Autodesk Fusion 360 part; units mm, degrees
(part 4 of 5)
  line L859 (16.6192, -17.6237) -> (17.4198, -17.6237)
  line L860 (17.4198, -17.6237) -> (17.4198, -20.7216)
  line L861 (17.4198, -20.7216) -> (16.6192, -20.7216)
  line L862 (16.6192, -20.7216) -> (16.6192, -21.722)
  line L863 (16.6192, -21.722) -> (2.6196, -21.722)
  line L864 (364.282, -27.7716) -> (365.083, -27.7716)
  line L865 (365.083, -27.7716) -> (365.083, -30.8722)
  line L866 (365.083, -30.8722) -> (364.282, -30.8722)
  line L867 (364.282, -30.8722) -> (364.282, -36.6737)
  line L868 (364.282, -36.6737) -> (365.083, -36.6737)
  line L869 (365.083, -36.6737) -> (365.083, -39.7715)
  line L870 (365.083, -39.7715) -> (364.282, -39.7715)
  line L871 (364.282, -39.7715) -> (364.282, -40.7719)
  line L872 (364.282, -40.7719) -> (350.282, -40.7719)
  line L873 (350.282, -40.7719) -> (350.282, -39.7715)
  line L874 (350.282, -39.7715) -> (349.481, -39.7715)
  line L875 (349.481, -39.7715) -> (349.481, -36.6737)
  line L876 (349.481, -36.6737) -> (350.282, -36.6737)
  line L877 (350.282, -36.6737) -> (350.282, -30.8722)
  line L878 (350.282, -30.8722) -> (349.481, -30.8722)
  line L879 (349.481, -30.8722) -> (349.481, -27.7716)
  line L880 (349.481, -27.7716) -> (350.282, -27.7716)
  line L881 (350.282, -27.7716) -> (350.282, -26.7725)
  line L882 (350.282, -26.7725) -> (364.282, -26.7725)
  line L883 (364.282, -26.7725) -> (364.282, -27.7716)
  line L884 (278.557, -39.7715) -> (278.557, -40.7719)
  line L885 (278.557, -40.7719) -> (264.557, -40.7719)
  line L886 (264.557, -40.7719) -> (264.557, -39.7715)
  line L887 (264.557, -39.7715) -> (263.756, -39.7715)
  line L888 (263.756, -39.7715) -> (263.756, -36.6737)
  line L889 (263.756, -36.6737) -> (264.557, -36.6737)
  line L890 (264.557, -36.6737) -> (264.557, -30.8722)
  line L891 (264.557, -30.8722) -> (263.756, -30.8722)
  line L892 (263.756, -30.8722) -> (263.756, -27.7716)
  line L893 (263.756, -27.7716) -> (264.557, -27.7716)
  line L894 (264.557, -27.7716) -> (264.557, -26.7725)
  line L895 (264.557, -26.7725) -> (278.557, -26.7725)
  line L896 (278.557, -26.7725) -> (278.557, -27.7716)
  line L897 (278.557, -27.7716) -> (279.356, -27.7716)
  line L898 (279.356, -27.7716) -> (279.356, -30.8722)
  line L899 (279.356, -30.8722) -> (278.557, -30.8722)
  line L900 (278.557, -30.8722) -> (278.557, -36.6737)
  line L901 (278.557, -36.6737) -> (279.356, -36.6737)
  line L902 (279.356, -36.6737) -> (279.356, -39.7715)
  line L903 (279.356, -39.7715) -> (278.557, -39.7715)
  line L904 (244.706, -36.6737) -> (245.507, -36.6737)
  line L905 (245.507, -36.6737) -> (245.507, -30.8722)
  line L906 (245.507, -30.8722) -> (244.706, -30.8722)
  line L907 (244.706, -30.8722) -> (244.706, -27.7716)
  line L908 (244.706, -27.7716) -> (245.507, -27.7716)
  line L909 (245.507, -27.7716) -> (245.507, -26.7725)
  line L910 (245.507, -26.7725) -> (259.507, -26.7725)
  line L911 (259.507, -26.7725) -> (259.507, -27.7716)
  line L912 (259.507, -27.7716) -> (260.306, -27.7716)
  line L913 (260.306, -27.7716) -> (260.306, -30.8722)
  line L914 (260.306, -30.8722) -> (259.507, -30.8722)
  line L915 (259.507, -30.8722) -> (259.507, -36.6737)
  line L916 (259.507, -36.6737) -> (260.306, -36.6737)
  line L917 (260.306, -36.6737) -> (260.306, -39.7715)
  line L918 (260.306, -39.7715) -> (259.507, -39.7715)
  line L919 (259.507, -39.7715) -> (259.507, -40.7719)
  line L920 (259.507, -40.7719) -> (245.507, -40.7719)
  line L921 (245.507, -40.7719) -> (245.507, -39.7715)
  line L922 (245.507, -39.7715) -> (244.706, -39.7715)
  line L923 (244.706, -39.7715) -> (244.706, -36.6737)
  line L924 (225.656, -30.8722) -> (225.656, -27.7716)
  line L925 (225.656, -27.7716) -> (226.457, -27.7716)
  line L926 (226.457, -27.7716) -> (226.457, -26.7725)
  line L927 (226.457, -26.7725) -> (240.457, -26.7725)
  line L928 (240.457, -26.7725) -> (240.457, -27.7716)
  line L929 (240.457, -27.7716) -> (241.256, -27.7716)
  line L930 (241.256, -27.7716) -> (241.256, -30.8722)
  line L931 (241.256, -30.8722) -> (240.457, -30.8722)
  line L932 (240.457, -30.8722) -> (240.457, -36.6737)
  line L933 (240.457, -36.6737) -> (241.256, -36.6737)
  line L934 (241.256, -36.6737) -> (241.256, -39.7715)
  line L935 (241.256, -39.7715) -> (240.457, -39.7715)
  line L936 (240.457, -39.7715) -> (240.457, -40.7719)
  line L937 (240.457, -40.7719) -> (226.457, -40.7719)
  line L938 (226.457, -40.7719) -> (226.457, -39.7715)
  line L939 (226.457, -39.7715) -> (225.656, -39.7715)
  line L940 (225.656, -39.7715) -> (225.656, -36.6737)
  line L941 (225.656, -36.6737) -> (226.457, -36.6737)
  line L942 (226.457, -36.6737) -> (226.457, -30.8722)
  line L943 (226.457, -30.8722) -> (225.656, -30.8722)
  line L944 (107.107, -40.7719) -> (93.1072, -40.7719)
  line L945 (93.1072, -40.7719) -> (93.1072, -39.7715)
  line L946 (93.1072, -39.7715) -> (92.3064, -39.7715)
  line L947 (92.3064, -39.7715) -> (92.3064, -36.6737)
  line L948 (92.3064, -36.6737) -> (93.1072, -36.6737)
  line L949 (93.1072, -36.6737) -> (93.1072, -30.8722)
  line L950 (93.1072, -30.8722) -> (92.3064, -30.8722)
  line L951 (92.3064, -30.8722) -> (92.3064, -27.7716)
  line L952 (92.3064, -27.7716) -> (93.1072, -27.7716)
  line L953 (93.1072, -27.7716) -> (93.1072, -26.7725)
  line L954 (93.1072, -26.7725) -> (107.107, -26.7725)
  line L955 (107.107, -26.7725) -> (107.107, -27.7716)
  line L956 (107.107, -27.7716) -> (107.906, -27.7716)
  line L957 (107.906, -27.7716) -> (107.906, -30.8722)
  line L958 (107.906, -30.8722) -> (107.107, -30.8722)
  line L959 (107.107, -30.8722) -> (107.107, -36.6737)
  line L960 (107.107, -36.6737) -> (107.906, -36.6737)
  line L961 (107.906, -36.6737) -> (107.906, -39.7715)
  line L962 (107.906, -39.7715) -> (107.107, -39.7715)
  line L963 (107.107, -39.7715) -> (107.107, -40.7719)
  line L964 (146.006, -39.7715) -> (145.207, -39.7715)
  line L965 (145.207, -39.7715) -> (145.207, -40.7719)
  line L966 (145.207, -40.7719) -> (131.207, -40.7719)
  line L967 (131.207, -40.7719) -> (131.207, -39.7715)
  line L968 (131.207, -39.7715) -> (130.406, -39.7715)
  line L969 (130.406, -39.7715) -> (130.406, -36.6737)
  line L970 (130.406, -36.6737) -> (131.207, -36.6737)
  line L971 (131.207, -36.6737) -> (131.207, -30.8722)
  line L972 (131.207, -30.8722) -> (130.406, -30.8722)
  line L973 (130.406, -30.8722) -> (130.406, -27.7716)
  line L974 (130.406, -27.7716) -> (131.207, -27.7716)
  line L975 (131.207, -27.7716) -> (131.207, -26.7725)
  line L976 (131.207, -26.7725) -> (145.207, -26.7725)
  line L977 (145.207, -26.7725) -> (145.207, -27.7716)
  line L978 (145.207, -27.7716) -> (146.006, -27.7716)
  line L979 (146.006, -27.7716) -> (146.006, -30.8722)
  line L980 (146.006, -30.8722) -> (145.207, -30.8722)
  line L981 (145.207, -30.8722) -> (145.207, -36.6737)
  line L982 (145.207, -36.6737) -> (146.006, -36.6737)
  line L983 (146.006, -36.6737) -> (146.006, -39.7715)
  line L984 (112.157, -36.6737) -> (112.157, -30.8722)
  line L985 (112.157, -30.8722) -> (111.356, -30.8722)
  line L986 (111.356, -30.8722) -> (111.356, -27.7716)
  line L987 (111.356, -27.7716) -> (112.157, -27.7716)
  line L988 (112.157, -27.7716) -> (112.157, -26.7725)
  line L989 (112.157, -26.7725) -> (126.157, -26.7725)
  line L990 (126.157, -26.7725) -> (126.157, -27.7716)
  line L991 (126.157, -27.7716) -> (126.956, -27.7716)
  line L992 (126.956, -27.7716) -> (126.956, -30.8722)
  line L993 (126.956, -30.8722) -> (126.157, -30.8722)
  line L994 (126.157, -30.8722) -> (126.157, -36.6737)
  line L995 (126.157, -36.6737) -> (126.956, -36.6737)
  line L996 (126.956, -36.6737) -> (126.956, -39.7715)
  line L997 (126.956, -39.7715) -> (126.157, -39.7715)
  line L998 (126.157, -39.7715) -> (126.157, -40.7719)
  line L999 (126.157, -40.7719) -> (112.157, -40.7719)
  line L1000 (112.157, -40.7719) -> (112.157, -39.7715)
  line L1001 (112.157, -39.7715) -> (111.356, -39.7715)
  line L1002 (111.356, -39.7715) -> (111.356, -36.6737)
  line L1003 (111.356, -36.6737) -> (112.157, -36.6737)
  line L1004 (36.4698, -36.6737) -> (36.4698, -39.7715)
  line L1005 (36.4698, -39.7715) -> (35.669, -39.7715)
  line L1006 (35.669, -39.7715) -> (35.669, -40.7719)
  line L1007 (35.669, -40.7719) -> (21.6697, -40.7719)
  line L1008 (21.6697, -40.7719) -> (21.6697, -39.7715)
  line L1009 (21.6697, -39.7715) -> (20.869, -39.7715)
  line L1010 (20.869, -39.7715) -> (20.869, -36.6737)
  line L1011 (20.869, -36.6737) -> (21.6697, -36.6737)
  line L1012 (21.6697, -36.6737) -> (21.6697, -30.8722)
  line L1013 (21.6697, -30.8722) -> (20.869, -30.8722)
  line L1014 (20.869, -30.8722) -> (20.869, -27.7716)
  line L1015 (20.869, -27.7716) -> (21.6697, -27.7716)
  line L1016 (21.6697, -27.7716) -> (21.6697, -26.7725)
  line L1017 (21.6697, -26.7725) -> (35.669, -26.7725)
  line L1018 (35.669, -26.7725) -> (35.669, -27.7716)
  line L1019 (35.669, -27.7716) -> (36.4698, -27.7716)
  line L1020 (36.4698, -27.7716) -> (36.4698, -30.8722)
  line L1021 (36.4698, -30.8722) -> (35.669, -30.8722)
  line L1022 (35.669, -30.8722) -> (35.669, -36.6737)
  line L1023 (35.669, -36.6737) -> (36.4698, -36.6737)
  line L1024 (16.6192, -40.7719) -> (2.6196, -40.7719)
  line L1025 (2.6197, -40.7719) -> (2.6197, -39.7715)
  line L1026 (2.6197, -39.7715) -> (1.819, -39.7715)
  line L1027 (1.819, -39.7715) -> (1.819, -36.6737)
  line L1028 (1.819, -36.6737) -> (2.6197, -36.6737)
  line L1029 (2.6197, -36.6737) -> (2.6197, -30.8722)
  line L1030 (2.6197, -30.8722) -> (1.819, -30.8722)
  line L1031 (1.819, -30.8722) -> (1.819, -27.7716)
  line L1032 (1.819, -27.7716) -> (2.6197, -27.7716)
  line L1033 (2.6197, -27.7716) -> (2.6197, -26.7725)
  line L1034 (2.6197, -26.7725) -> (16.6192, -26.7725)
  line L1035 (16.6192, -26.7725) -> (16.6192, -27.7716)
  line L1036 (16.6192, -27.7716) -> (17.4198, -27.7716)
  line L1037 (17.4198, -27.7716) -> (17.4198, -30.8722)
  line L1038 (17.4198, -30.8722) -> (16.6192, -30.8722)
  line L1039 (16.6192, -30.8722) -> (16.6192, -36.6737)
  line L1040 (16.6192, -36.6737) -> (17.4198, -36.6737)
  line L1041 (17.4198, -36.6737) -> (17.4198, -39.7715)
  line L1042 (17.4198, -39.7715) -> (16.6192, -39.7715)
  line L1043 (16.6192, -39.7715) -> (16.6192, -40.7719)
  line L1044 (349.481, -46.8217) -> (350.282, -46.8217)
  line L1045 (350.282, -46.8217) -> (350.282, -45.8227)
  line L1046 (350.282, -45.8227) -> (364.282, -45.8227)
  line L1047 (364.282, -45.8227) -> (364.282, -46.8217)
  line L1048 (364.282, -46.8217) -> (365.083, -46.8217)
  line L1049 (365.083, -46.8217) -> (365.083, -49.9223)
  line L1050 (365.083, -49.9223) -> (364.282, -49.9223)
  line L1051 (364.282, -49.9223) -> (364.282, -55.7223)
  line L1052 (364.282, -55.7223) -> (365.083, -55.7223)
  line L1053 (365.083, -55.7223) -> (365.083, -58.8215)
  line L1054 (365.083, -58.8215) -> (364.282, -58.8215)
  line L1055 (364.282, -58.8215) -> (364.282, -59.8219)
  line L1056 (364.282, -59.8219) -> (350.282, -59.8219)
  line L1057 (350.282, -59.8219) -> (350.282, -58.8215)
  line L1058 (350.282, -58.8215) -> (349.481, -58.8215)
  line L1059 (349.481, -58.8215) -> (349.481, -55.7223)
  line L1060 (349.481, -55.7223) -> (350.282, -55.7223)
  line L1061 (350.282, -55.7223) -> (350.282, -49.9223)
  line L1062 (350.282, -49.9223) -> (349.481, -49.9223)
  line L1063 (349.481, -49.9223) -> (349.481, -46.8217)
  line L1064 (288.082, -59.8219) -> (274.082, -59.8219)
  line L1065 (274.082, -59.8219) -> (274.082, -58.8215)
  line L1066 (274.082, -58.8215) -> (273.281, -58.8215)
  line L1067 (273.281, -58.8215) -> (273.281, -55.7223)
  line L1068 (273.281, -55.7223) -> (274.082, -55.7223)
  line L1069 (274.082, -55.7223) -> (274.082, -49.9223)
  line L1070 (274.082, -49.9223) -> (273.281, -49.9223)
  line L1071 (273.281, -49.9223) -> (273.281, -46.8217)
  line L1072 (273.281, -46.8217) -> (274.082, -46.8217)
  line L1073 (274.082, -46.8217) -> (274.082, -45.8227)
  line L1074 (274.082, -45.8227) -> (288.082, -45.8227)
  line L1075 (288.082, -45.8227) -> (288.082, -46.8217)
  line L1076 (288.082, -46.8217) -> (288.881, -46.8217)
  line L1077 (288.881, -46.8217) -> (288.881, -49.9223)
  line L1078 (288.881, -49.9223) -> (288.082, -49.9223)
  line L1079 (288.082, -49.9223) -> (288.082, -55.7223)
  line L1080 (288.082, -55.7223) -> (288.881, -55.7223)
  line L1081 (288.881, -55.7223) -> (288.881, -58.8215)
  line L1082 (288.881, -58.8215) -> (288.082, -58.8215)
  line L1083 (288.082, -58.8215) -> (288.082, -59.8219)
  line L1084 (249.982, -55.7223) -> (250.781, -55.7223)
  line L1085 (250.781, -55.7223) -> (250.781, -58.8215)
  line L1086 (250.781, -58.8215) -> (249.982, -58.8215)
  line L1087 (249.982, -58.8215) -> (249.982, -59.8219)
  line L1088 (249.982, -59.8219) -> (235.982, -59.8219)
  line L1089 (235.982, -59.8219) -> (235.982, -58.8215)
  line L1090 (235.982, -58.8215) -> (235.181, -58.8215)
  line L1091 (235.181, -58.8215) -> (235.181, -55.7223)
  line L1092 (235.181, -55.7223) -> (235.982, -55.7223)
  line L1093 (235.982, -55.7223) -> (235.982, -49.9223)
  line L1094 (235.982, -49.9223) -> (235.181, -49.9223)
  line L1095 (235.181, -49.9223) -> (235.181, -46.8217)
  line L1096 (235.181, -46.8217) -> (235.982, -46.8217)
  line L1097 (235.982, -46.8217) -> (235.982, -45.8227)
  line L1098 (235.982, -45.8227) -> (249.982, -45.8227)
  line L1099 (249.982, -45.8227) -> (249.982, -46.8217)
  line L1100 (249.982, -46.8217) -> (250.781, -46.8217)
  line L1101 (250.781, -46.8217) -> (250.781, -49.9223)
  line L1102 (250.781, -49.9223) -> (249.982, -49.9223)
  line L1103 (249.982, -49.9223) -> (249.982, -55.7223)
  line L1104 (269.032, -46.8217) -> (269.831, -46.8217)
  line L1105 (269.831, -46.8217) -> (269.831, -49.9223)
  line L1106 (269.831, -49.9223) -> (269.032, -49.9223)
  line L1107 (269.032, -49.9223) -> (269.032, -55.7223)
  line L1108 (269.032, -55.7223) -> (269.831, -55.7223)
  line L1109 (269.831, -55.7223) -> (269.831, -58.8215)
  line L1110 (269.831, -58.8215) -> (269.032, -58.8215)
  line L1111 (269.032, -58.8215) -> (269.032, -59.8219)
  line L1112 (269.032, -59.8219) -> (255.032, -59.8219)
  line L1113 (255.032, -59.8219) -> (255.032, -58.8215)
  line L1114 (255.032, -58.8215) -> (254.231, -58.8215)
  line L1115 (254.231, -58.8215) -> (254.231, -55.7223)
  line L1116 (254.231, -55.7223) -> (255.032, -55.7223)
  line L1117 (255.032, -55.7223) -> (255.032, -49.9223)
  line L1118 (255.032, -49.9223) -> (254.231, -49.9223)
  line L1119 (254.231, -49.9223) -> (254.231, -46.8217)
  line L1120 (254.231, -46.8217) -> (255.032, -46.8217)
  line L1121 (255.032, -46.8217) -> (255.032, -45.8227)
  line L1122 (255.032, -45.8227) -> (269.032, -45.8227)
  line L1123 (269.032, -45.8227) -> (269.032, -46.8217)
  line L1124 (230.932, -45.8227) -> (230.932, -46.8217)
  line L1125 (230.932, -46.8217) -> (231.731, -46.8217)
  line L1126 (231.731, -46.8217) -> (231.731, -49.9223)
  line L1127 (231.731, -49.9223) -> (230.932, -49.9223)
  line L1128 (230.932, -49.9223) -> (230.932, -55.7223)
  line L1129 (230.932, -55.7223) -> (231.731, -55.7223)
  line L1130 (231.731, -55.7223) -> (231.731, -58.8215)
  line L1131 (231.731, -58.8215) -> (230.932, -58.8215)
  line L1132 (230.932, -58.8215) -> (230.932, -59.8219)
  line L1133 (230.932, -59.8219) -> (216.932, -59.8219)
  line L1134 (216.932, -59.8219) -> (216.932, -58.8215)
  line L1135 (216.932, -58.8215) -> (216.131, -58.8215)
  line L1136 (216.131, -58.8215) -> (216.131, -55.7223)
  line L1137 (216.131, -55.7223) -> (216.932, -55.7223)
  line L1138 (216.932, -55.7223) -> (216.932, -49.9223)
  line L1139 (216.932, -49.9223) -> (216.131, -49.9223)
  line L1140 (216.131, -49.9223) -> (216.131, -46.8217)
  line L1141 (216.131, -46.8217) -> (216.932, -46.8217)
  line L1142 (216.932, -46.8217) -> (216.932, -45.8227)
  line L1143 (216.932, -45.8227) -> (230.932, -45.8227)
  line L1144 (174.581, -46.8217) -> (174.581, -49.9223)
  line L1145 (174.581, -49.9223) -> (173.782, -49.9223)
  line L1146 (173.782, -49.9223) -> (173.782, -55.7223)
  line L1147 (173.782, -55.7223) -> (174.581, -55.7223)
  line L1148 (174.581, -55.7223) -> (174.581, -58.8215)
  line L1149 (174.581, -58.8215) -> (173.782, -58.8215)
  line L1150 (173.782, -58.8215) -> (173.782, -59.8219)
  line L1151 (173.782, -59.8219) -> (159.782, -59.8219)
  line L1152 (159.782, -59.8219) -> (159.782, -58.8215)
  line L1153 (159.782, -58.8215) -> (158.981, -58.8215)
  line L1154 (158.981, -58.8215) -> (158.981, -55.7223)
  line L1155 (158.981, -55.7223) -> (159.782, -55.7223)
  line L1156 (159.782, -55.7223) -> (159.782, -49.9223)
  line L1157 (159.782, -49.9223) -> (158.981, -49.9223)
  line L1158 (158.981, -49.9223) -> (158.981, -46.8217)
  line L1159 (158.981, -46.8217) -> (159.782, -46.8217)
  line L1160 (159.782, -46.8217) -> (159.782, -45.8227)
  line L1161 (159.782, -45.8227) -> (173.782, -45.8227)
  line L1162 (173.782, -45.8227) -> (173.782, -46.8217)
  line L1163 (173.782, -46.8217) -> (174.581, -46.8217)
  line L1164 (211.882, -49.9223) -> (211.882, -55.7223)
  line L1165 (211.882, -55.7223) -> (212.681, -55.7223)
  line L1166 (212.681, -55.7223) -> (212.681, -58.8215)
  line L1167 (212.681, -58.8215) -> (211.882, -58.8215)
  line L1168 (211.882, -58.8215) -> (211.882, -59.8219)
  line L1169 (211.882, -59.8219) -> (197.882, -59.8219)
  line L1170 (197.882, -59.8219) -> (197.882, -58.8215)
  line L1171 (197.882, -58.8215) -> (197.081, -58.8215)
  line L1172 (197.081, -58.8215) -> (197.081, -55.7223)
  line L1173 (197.081, -55.7223) -> (197.882, -55.7223)
  line L1174 (197.882, -55.7223) -> (197.882, -49.9223)
  line L1175 (197.882, -49.9223) -> (197.081, -49.9223)
  line L1176 (197.081, -49.9223) -> (197.081, -46.8217)
  line L1177 (197.081, -46.8217) -> (197.882, -46.8217)
  line L1178 (197.882, -46.8217) -> (197.882, -45.8227)
  line L1179 (197.882, -45.8227) -> (211.882, -45.8227)
  line L1180 (211.882, -45.8227) -> (211.882, -46.8217)
  line L1181 (211.882, -46.8217) -> (212.681, -46.8217)
  line L1182 (212.681, -46.8217) -> (212.681, -49.9223)
  line L1183 (212.681, -49.9223) -> (211.882, -49.9223)
  line L1184 (109.488, -8.7216) -> (110.287, -8.7216)
  line L1185 (110.287, -8.7216) -> (110.287, -11.8222)
  line L1186 (110.287, -11.8222) -> (109.488, -11.8222)
  line L1187 (109.488, -11.8222) -> (109.488, -17.6237)
  line L1188 (109.488, -17.6237) -> (110.287, -17.6237)
  line L1189 (110.287, -17.6237) -> (110.287, -20.7216)
  line L1190 (110.287, -20.7216) -> (109.488, -20.7216)
  line L1191 (109.488, -20.7216) -> (109.488, -21.722)
  line L1192 (109.488, -21.722) -> (95.4871, -21.722)
  line L1193 (95.4871, -21.722) -> (95.4871, -20.7216)
  line L1194 (95.4871, -20.7216) -> (94.6877, -20.7216)
  line L1195 (94.6877, -20.7216) -> (94.6877, -17.6237)
  line L1196 (94.6877, -17.6237) -> (95.4871, -17.6237)
  line L1197 (95.4871, -17.6237) -> (95.4871, -11.8222)
  line L1198 (95.4871, -11.8222) -> (94.6877, -11.8222)
  line L1199 (94.6877, -11.8222) -> (94.6877, -8.7216)
  line L1200 (94.6877, -8.7216) -> (95.4871, -8.7216)
  line L1201 (95.4871, -8.7216) -> (95.4871, -7.7225)
  line L1202 (95.4871, -7.7225) -> (109.488, -7.7225)
  line L1203 (109.488, -7.7225) -> (109.488, -8.7216)
  line L1204 (253.162, -11.8222) -> (252.361, -11.8222)
  line L1205 (252.361, -11.8222) -> (252.361, -17.6237)
  line L1206 (252.361, -17.6237) -> (253.162, -17.6237)
  line L1207 (253.162, -17.6237) -> (253.162, -20.7216)
  line L1208 (253.162, -20.7216) -> (252.361, -20.7216)
  line L1209 (252.361, -20.7216) -> (252.361, -21.722)
  line L1210 (252.361, -21.722) -> (238.362, -21.722)
  line L1211 (238.362, -21.722) -> (238.362, -20.7216)
  line L1212 (238.362, -20.7216) -> (237.563, -20.7216)
  line L1213 (237.563, -20.7216) -> (237.563, -17.6237)
  line L1214 (237.563, -17.6237) -> (238.362, -17.6237)
  line L1215 (238.362, -17.6237) -> (238.362, -11.8222)
  line L1216 (238.362, -11.8222) -> (237.563, -11.8222)
  line L1217 (237.563, -11.8222) -> (237.563, -8.7216)
  line L1218 (237.563, -8.7216) -> (238.362, -8.7216)
  line L1219 (238.362, -8.7216) -> (238.362, -7.7225)
  line L1220 (238.362, -7.7225) -> (252.361, -7.7225)
  line L1221 (252.361, -7.7225) -> (252.361, -8.7216)
  line L1222 (252.361, -8.7216) -> (253.162, -8.7216)
  line L1223 (253.162, -8.7216) -> (253.162, -11.8222)
  line L1224 (52.626, -8.7216) -> (52.626, -7.7225)
  line L1225 (52.626, -7.7225) -> (66.6253, -7.7225)
  line L1226 (66.6253, -7.7225) -> (66.6253, -8.7216)
  line L1227 (66.6253, -8.7216) -> (67.4261, -8.7216)
  line L1228 (67.4261, -8.7216) -> (67.4261, -11.8222)
  line L1229 (67.4261, -11.8222) -> (66.6253, -11.8222)
  line L1230 (66.6253, -11.8222) -> (66.6253, -17.6237)
  line L1231 (66.6253, -17.6237) -> (67.4261, -17.6237)
  line L1232 (67.4261, -17.6237) -> (67.4261, -20.7216)
  line L1233 (67.4261, -20.7216) -> (66.6253, -20.7216)
  line L1234 (66.6253, -20.7216) -> (66.6253, -21.722)
  line L1235 (66.6253, -21.722) -> (52.626, -21.722)
  line L1236 (52.626, -21.722) -> (52.626, -20.7216)
  line L1237 (52.626, -20.7216) -> (51.8252, -20.7216)
  line L1238 (51.8252, -20.7216) -> (51.8252, -17.6237)
  line L1239 (51.8252, -17.6237) -> (52.626, -17.6237)
  line L1240 (52.626, -17.6237) -> (52.626, -11.8222)
  line L1241 (52.626, -11.8222) -> (51.8252, -11.8222)
  line L1242 (51.8252, -11.8222) -> (51.8252, -8.7216)
  line L1243 (51.8252, -8.7216) -> (52.626, -8.7216)
  line L1244 (21.6697, -21.722) -> (21.6697, -20.7216)
  line L1245 (21.6697, -20.7216) -> (20.869, -20.7216)
  line L1246 (20.869, -20.7216) -> (20.869, -17.6237)
  line L1247 (20.869, -17.6237) -> (21.6697, -17.6237)
  line L1248 (21.6697, -17.6237) -> (21.6697, -11.8222)
  line L1249 (21.6697, -11.8222) -> (20.869, -11.8222)
  line L1250 (20.869, -11.8222) -> (20.869, -8.7216)
  line L1251 (20.869, -8.7216) -> (21.6697, -8.7216)
  line L1252 (21.6697, -8.7216) -> (21.6697, -7.7225)
  line L1253 (21.6697, -7.7225) -> (35.669, -7.7225)
  line L1254 (35.669, -7.7225) -> (35.669, -8.7216)
  line L1255 (35.669, -8.7216) -> (36.4698, -8.7216)
  line L1256 (36.4698, -8.7216) -> (36.4698, -11.8222)
  line L1257 (36.4698, -11.8222) -> (35.669, -11.8222)
  line L1258 (35.669, -11.8222) -> (35.669, -17.6237)
  line L1259 (35.669, -17.6237) -> (36.4698, -17.6237)
  line L1260 (36.4698, -17.6237) -> (36.4698, -20.7216)
  line L1261 (36.4698, -20.7216) -> (35.669, -20.7216)
  line L1262 (35.669, -20.7216) -> (35.669, -21.722)
  line L1263 (35.669, -21.722) -> (21.6697, -21.722)
  line L1264 (295.225, -11.8222) -> (295.225, -17.6237)
  line L1265 (295.225, -17.6237) -> (296.026, -17.6237)
  line L1266 (296.026, -17.6237) -> (296.026, -20.7216)
  line L1267 (296.026, -20.7216) -> (295.225, -20.7216)
  line L1268 (295.225, -20.7216) -> (295.225, -21.722)
  line L1269 (295.225, -21.722) -> (281.226, -21.722)
  line L1270 (281.226, -21.722) -> (281.226, -20.7216)
  line L1271 (281.226, -20.7216) -> (280.425, -20.7216)
  line L1272 (280.425, -20.7216) -> (280.425, -17.6237)
  line L1273 (280.425, -17.6237) -> (281.226, -17.6237)
  line L1274 (281.226, -17.6237) -> (281.226, -11.8222)
  line L1275 (281.226, -11.8222) -> (280.425, -11.8222)
  line L1276 (280.425, -11.8222) -> (280.425, -8.7216)
  line L1277 (280.425, -8.7216) -> (281.226, -8.7216)
  line L1278 (281.226, -8.7216) -> (281.226, -7.7225)
  line L1279 (281.226, -7.7225) -> (295.225, -7.7225)
  line L1280 (295.225, -7.7225) -> (295.225, -8.7216)
  line L1281 (295.225, -8.7216) -> (296.026, -8.7216)
  line L1282 (296.026, -8.7216) -> (296.026, -11.8222)
  line L1283 (296.026, -11.8222) -> (295.225, -11.8222)
  line L1284 (321.419, -3.9605) -> (322.22, -3.9605)
  line L1285 (322.22, -3.9605) -> (322.22, -7.0597)
  line L1286 (322.22, -7.0597) -> (321.419, -7.0597)
  line L1287 (321.419, -7.0597) -> (321.419, -12.8598)
  line L1288 (321.419, -12.8598) -> (322.22, -12.8598)
  line L1289 (322.22, -12.8598) -> (322.22, -15.9604)
  line L1290 (322.22, -15.9604) -> (321.419, -15.9604)
  line L1291 (321.419, -15.9604) -> (321.419, -16.9595)
  line L1292 (321.419, -16.9595) -> (307.42, -16.9595)
  line L1293 (307.42, -16.9595) -> (307.42, -15.9604)
  line L1294 (307.42, -15.9604) -> (306.619, -15.9604)
  line L1295 (306.619, -15.9604) -> (306.619, -12.8598)
  line L1296 (306.619, -12.8598) -> (307.42, -12.8598)
  line L1297 (307.42, -12.8598) -> (307.42, -7.0597)
  line L1298 (307.42, -7.0597) -> (306.619, -7.0597)
  line L1299 (306.619, -7.0597) -> (306.619, -3.9605)
  line L1300 (306.619, -3.9605) -> (307.42, -3.9605)
  line L1301 (307.42, -3.9605) -> (307.42, -2.96)
  line L1302 (307.42, -2.96) -> (321.419, -2.96)
  line L1303 (321.419, -2.96) -> (321.419, -3.9605)
  line L1304 (84.0948, -93.8223) -> (84.0948, -96.9215)
  line L1305 (84.0948, -96.9215) -> (83.294, -96.9215)
  line L1306 (83.294, -96.9215) -> (83.294, -97.9219)
  line L1307 (83.294, -97.9219) -> (69.2947, -97.9219)
  line L1308 (69.2947, -97.9219) -> (69.2947, -96.9215)
  line L1309 (69.2947, -96.9215) -> (68.4939, -96.9215)
  line L1310 (68.4939, -96.9215) -> (68.4939, -93.8223)
  line L1311 (68.4939, -93.8223) -> (69.2947, -93.8223)
  line L1312 (69.2947, -93.8223) -> (69.2947, -88.0223)
  line L1313 (69.2947, -88.0223) -> (68.4939, -88.0223)
  line L1314 (68.4939, -88.0223) -> (68.4939, -84.9217)
  line L1315 (68.4939, -84.9217) -> (69.2947, -84.9217)
  line L1316 (69.2947, -84.9217) -> (69.2947, -83.9227)
  line L1317 (69.2947, -83.9227) -> (83.294, -83.9227)
  line L1318 (83.294, -83.9227) -> (83.294, -84.9217)
  line L1319 (83.294, -84.9217) -> (84.0948, -84.9217)
  line L1320 (84.0948, -84.9217) -> (84.0948, -88.0223)
  line L1321 (84.0948, -88.0223) -> (83.294, -88.0223)
  line L1322 (83.294, -88.0223) -> (83.294, -93.8223)
  line L1323 (83.294, -93.8223) -> (84.0948, -93.8223)
  line L1324 (102.344, -84.9217) -> (103.145, -84.9217)
  line L1325 (103.145, -84.9217) -> (103.145, -88.0223)
  line L1326 (103.145, -88.0223) -> (102.344, -88.0223)
  line L1327 (102.344, -88.0223) -> (102.344, -93.8223)
  line L1328 (102.344, -93.8223) -> (103.145, -93.8223)
  line L1329 (103.145, -93.8223) -> (103.145, -96.9215)
  line L1330 (103.145, -96.9215) -> (102.344, -96.9215)
  line L1331 (102.344, -96.9215) -> (102.344, -97.9219)
  line L1332 (102.344, -97.9219) -> (88.3447, -97.9219)
  line L1333 (88.3447, -97.9219) -> (88.3447, -96.9215)
  line L1334 (88.3447, -96.9215) -> (87.5439, -96.9215)
  line L1335 (87.5439, -96.9215) -> (87.5439, -93.8223)
  line L1336 (87.5439, -93.8223) -> (88.3447, -93.8223)
  line L1337 (88.3447, -93.8223) -> (88.3447, -88.0223)
  line L1338 (88.3447, -88.0223) -> (87.5439, -88.0223)
  line L1339 (87.5439, -88.0223) -> (87.5439, -84.9217)
  line L1340 (87.5439, -84.9217) -> (88.3447, -84.9217)
  line L1341 (88.3447, -84.9217) -> (88.3447, -83.9227)
  line L1342 (88.3447, -83.9227) -> (102.344, -83.9227)
  line L1343 (102.344, -83.9227) -> (102.344, -84.9217)
  line L1344 (107.395, -84.9217) -> (107.395, -83.9227)
  line L1345 (107.395, -83.9227) -> (121.394, -83.9227)
  line L1346 (121.394, -83.9227) -> (121.394, -84.9217)
  line L1347 (121.394, -84.9217) -> (122.195, -84.9217)
  line L1348 (122.195, -84.9217) -> (122.195, -88.0223)
  line L1349 (122.195, -88.0223) -> (121.394, -88.0223)
  line L1350 (121.394, -88.0223) -> (121.394, -93.8223)
  line L1351 (121.394, -93.8223) -> (122.195, -93.8223)
  line L1352 (122.195, -93.8223) -> (122.195, -96.9215)
  line L1353 (122.195, -96.9215) -> (121.394, -96.9215)
  line L1354 (121.394, -96.9215) -> (121.394, -97.9219)
  line L1355 (121.394, -97.9219) -> (107.395, -97.9219)
  line L1356 (107.395, -97.9219) -> (107.395, -96.9215)
  line L1357 (107.395, -96.9215) -> (106.594, -96.9215)
  line L1358 (106.594, -96.9215) -> (106.594, -93.8223)
  line L1359 (106.594, -93.8223) -> (107.395, -93.8223)
  line L1360 (107.395, -93.8223) -> (107.395, -88.0223)
  line L1361 (107.395, -88.0223) -> (106.594, -88.0223)
  line L1362 (106.594, -88.0223) -> (106.594, -84.9217)
  line L1363 (106.594, -84.9217) -> (107.395, -84.9217)
  line L1364 (2.6197, -83.9227) -> (16.6192, -83.9227)
  line L1365 (16.6192, -83.9227) -> (16.6192, -84.9217)
  line L1366 (16.6192, -84.9217) -> (17.4198, -84.9217)
  line L1367 (17.4198, -84.9217) -> (17.4198, -88.0223)
  line L1368 (17.4198, -88.0223) -> (16.6192, -88.0223)
  line L1369 (16.6192, -88.0223) -> (16.6192, -93.8223)
  line L1370 (16.6192, -93.8223) -> (17.4198, -93.8223)
  line L1371 (17.4198, -93.8223) -> (17.4198, -96.9215)
  line L1372 (17.4198, -96.9215) -> (16.6192, -96.9215)
  line L1373 (16.6192, -96.9215) -> (16.6192, -97.9219)
  line L1374 (16.6192, -97.9219) -> (2.6196, -97.9219)
  line L1375 (2.6197, -97.9219) -> (2.6197, -96.9215)
  line L1376 (2.6197, -96.9215) -> (1.819, -96.9215)
  line L1377 (1.819, -96.9215) -> (1.819, -93.8223)
  line L1378 (1.819, -93.8223) -> (2.6197, -93.8223)
  line L1379 (2.6197, -93.8223) -> (2.6197, -88.0223)
  line L1380 (2.6197, -88.0223) -> (1.819, -88.0223)
  line L1381 (1.819, -88.0223) -> (1.819, -84.9217)
  line L1382 (1.819, -84.9217) -> (2.6197, -84.9217)
  line L1383 (2.6197, -84.9217) -> (2.6197, -83.9227)
  line L1384 (50.2447, -97.9219) -> (50.2447, -96.9215)
  line L1385 (50.2447, -96.9215) -> (49.4439, -96.9215)
  line L1386 (49.4439, -96.9215) -> (49.4439, -93.8223)
  line L1387 (49.4439, -93.8223) -> (50.2447, -93.8223)
  line L1388 (50.2447, -93.8223) -> (50.2447, -88.0223)
  line L1389 (50.2447, -88.0223) -> (49.4439, -88.0223)
  line L1390 (49.4439, -88.0223) -> (49.4439, -84.9217)
  line L1391 (49.4439, -84.9217) -> (50.2447, -84.9217)
  line L1392 (50.2447, -84.9217) -> (50.2447, -83.9227)
  line L1393 (50.2447, -83.9227) -> (64.244, -83.9227)
  line L1394 (64.244, -83.9227) -> (64.244, -84.9217)
  line L1395 (64.244, -84.9217) -> (65.0448, -84.9217)
  line L1396 (65.0448, -84.9217) -> (65.0448, -88.0223)
  line L1397 (65.0448, -88.0223) -> (64.244, -88.0223)
  line L1398 (64.244, -88.0223) -> (64.244, -93.8223)
  line L1399 (64.244, -93.8223) -> (65.0448, -93.8223)
  line L1400 (65.0448, -93.8223) -> (65.0448, -96.9215)
  line L1401 (65.0448, -96.9215) -> (64.244, -96.9215)
  line L1402 (64.244, -96.9215) -> (64.244, -97.9219)
  line L1403 (64.244, -97.9219) -> (50.2447, -97.9219)
  line L1404 (21.6697, -93.8223) -> (21.6697, -88.0223)
  line L1405 (21.6697, -88.0223) -> (20.869, -88.0223)
  line L1406 (20.869, -88.0223) -> (20.869, -84.9217)
  line L1407 (20.869, -84.9217) -> (21.6697, -84.9217)
  line L1408 (21.6697, -84.9217) -> (21.6697, -83.9227)
  line L1409 (21.6697, -83.9227) -> (35.669, -83.9227)
  line L1410 (35.669, -83.9227) -> (35.669, -84.9217)
  line L1411 (35.669, -84.9217) -> (36.4698, -84.9217)
  line L1412 (36.4698, -84.9217) -> (36.4698, -88.0223)
  line L1413 (36.4698, -88.0223) -> (35.669, -88.0223)
  line L1414 (35.669, -88.0223) -> (35.669, -93.8223)
  line L1415 (35.669, -93.8223) -> (36.4698, -93.8223)
  line L1416 (36.4698, -93.8223) -> (36.4698, -96.9215)
  line L1417 (36.4698, -96.9215) -> (35.669, -96.9215)
  line L1418 (35.669, -96.9215) -> (35.669, -97.9219)
  line L1419 (35.669, -97.9219) -> (21.6697, -97.9219)
  line L1420 (21.6697, -97.9219) -> (21.6697, -96.9215)
  line L1421 (21.6697, -96.9215) -> (20.869, -96.9215)
  line L1422 (20.869, -96.9215) -> (20.869, -93.8223)
  line L1423 (20.869, -93.8223) -> (21.6697, -93.8223)
  line L1424 (140.444, -88.0223) -> (140.444, -93.8223)
  line L1425 (140.444, -93.8223) -> (141.245, -93.8223)
  line L1426 (141.245, -93.8223) -> (141.245, -96.9215)
  line L1427 (141.245, -96.9215) -> (140.444, -96.9215)
  line L1428 (140.444, -96.9215) -> (140.444, -97.9219)
  line L1429 (140.444, -97.9219) -> (126.445, -97.9219)
  line L1430 (126.445, -97.9219) -> (126.445, -96.9215)
  line L1431 (126.445, -96.9215) -> (125.644, -96.9215)
  line L1432 (125.644, -96.9215) -> (125.644, -93.8223)
  line L1433 (125.644, -93.8223) -> (126.445, -93.8223)
  line L1434 (126.445, -93.8223) -> (126.445, -88.0223)
  line L1435 (126.445, -88.0223) -> (125.644, -88.0223)
  line L1436 (125.644, -88.0223) -> (125.644, -84.9217)
  line L1437 (125.644, -84.9217) -> (126.445, -84.9217)
  line L1438 (126.445, -84.9217) -> (126.445, -83.9227)
  line L1439 (126.445, -83.9227) -> (140.444, -83.9227)
  line L1440 (140.444, -83.9227) -> (140.444, -84.9217)
  line L1441 (140.444, -84.9217) -> (141.245, -84.9217)
  line L1442 (141.245, -84.9217) -> (141.245, -88.0223)
  line L1443 (141.245, -88.0223) -> (140.444, -88.0223)
  line L1444 (2.6197, -55.7223) -> (2.6197, -49.9223)
  line L1445 (2.6197, -49.9223) -> (1.819, -49.9223)
  line L1446 (1.819, -49.9223) -> (1.819, -46.8217)
  line L1447 (1.819, -46.8217) -> (2.6197, -46.8217)
  line L1448 (2.6197, -46.8217) -> (2.6197, -45.8227)
  line L1449 (2.6197, -45.8227) -> (16.6192, -45.8227)
  line L1450 (16.6192, -45.8227) -> (16.6192, -46.8217)
  line L1451 (16.6192, -46.8217) -> (17.4198, -46.8217)
  line L1452 (17.4198, -46.8217) -> (17.4198, -49.9223)
  line L1453 (17.4198, -49.9223) -> (16.6192, -49.9223)
  line L1454 (16.6192, -49.9223) -> (16.6192, -55.7223)
  line L1455 (16.6192, -55.7223) -> (17.4198, -55.7223)
  line L1456 (17.4198, -55.7223) -> (17.4198, -58.8215)
  line L1457 (17.4198, -58.8215) -> (16.6192, -58.8215)
  line L1458 (16.6192, -58.8215) -> (16.6192, -59.8219)
  line L1459 (16.6192, -59.8219) -> (2.6196, -59.8219)
  line L1460 (2.6197, -59.8219) -> (2.6197, -58.8215)
  line L1461 (2.6197, -58.8215) -> (1.819, -58.8215)
  line L1462 (1.819, -58.8215) -> (1.819, -55.7223)
  line L1463 (1.819, -55.7223) -> (2.6197, -55.7223)
  line L1464 (312.182, -78.8719) -> (312.182, -77.8715)
  line L1465 (312.182, -77.8715) -> (311.381, -77.8715)
  line L1466 (311.381, -77.8715) -> (311.381, -74.7723)
  line L1467 (311.381, -74.7723) -> (312.182, -74.7723)
  line L1468 (312.182, -74.7723) -> (312.182, -68.9723)
  line L1469 (312.182, -68.9723) -> (311.381, -68.9723)
  line L1470 (311.381, -68.9723) -> (311.381, -65.8717)
  line L1471 (311.381, -65.8717) -> (312.182, -65.8717)
  line L1472 (312.182, -65.8717) -> (312.182, -64.8727)
  line L1473 (312.182, -64.8727) -> (326.182, -64.8727)
  line L1474 (326.182, -64.8727) -> (326.182, -65.8717)
  line L1475 (326.182, -65.8717) -> (326.981, -65.8717)
  line L1476 (326.981, -65.8717) -> (326.981, -68.9723)
  line L1477 (326.981, -68.9723) -> (326.182, -68.9723)
  line L1478 (326.182, -68.9723) -> (326.182, -74.7723)
  line L1479 (326.182, -74.7723) -> (326.981, -74.7723)
  line L1480 (326.981, -74.7723) -> (326.981, -77.8715)
  line L1481 (326.981, -77.8715) -> (326.182, -77.8715)
  line L1482 (326.182, -77.8715) -> (326.182, -78.8719)
  line L1483 (326.182, -78.8719) -> (312.182, -78.8719)
  line L1484 (71.3878, -55.7223) -> (72.1872, -55.7223)
  line L1485 (72.1872, -55.7223) -> (72.1872, -58.8215)
  line L1486 (72.1872, -58.8215) -> (71.3878, -58.8215)
  line L1487 (71.3878, -58.8215) -> (71.3878, -59.8219)
  line L1488 (71.3878, -59.8219) -> (52.626, -59.8219)
  line L1489 (52.626, -59.8219) -> (52.626, -58.8215)
  line L1490 (52.626, -58.8215) -> (51.8252, -58.8215)
  line L1491 (51.8252, -58.8215) -> (51.8252, -55.7223)
  line L1492 (51.8252, -55.7223) -> (52.626, -55.7223)
  line L1493 (52.626, -55.7223) -> (52.626, -49.9223)
  line L1494 (52.626, -49.9223) -> (51.8252, -49.9223)
  line L1495 (51.8252, -49.9223) -> (51.8252, -46.8217)
  line L1496 (51.8252, -46.8217) -> (52.626, -46.8217)
  line L1497 (52.626, -46.8217) -> (52.626, -45.8227)
  line L1498 (52.626, -45.8227) -> (71.3878, -45.8227)
  line L1499 (71.3878, -45.8227) -> (71.3878, -46.8217)
  line L1500 (71.3878, -46.8217) -> (72.1872, -46.8217)
  line L1501 (72.1872, -46.8217) -> (72.1872, -49.9223)
  line L1502 (72.1872, -49.9223) -> (71.3878, -49.9223)
  line L1503 (71.3878, -49.9223) -> (71.3878, -55.7223)
  line L1504 (21.6697, -59.8219) -> (21.6697, -58.8215)
  line L1505 (21.6697, -58.8215) -> (20.869, -58.8215)
  line L1506 (20.869, -58.8215) -> (20.869, -55.7223)
  line L1507 (20.869, -55.7223) -> (21.6697, -55.7223)
  line L1508 (21.6697, -55.7223) -> (21.6697, -49.9223)
  line L1509 (21.6697, -49.9223) -> (20.869, -49.9223)
  line L1510 (20.869, -49.9223) -> (20.869, -46.8217)
  line L1511 (20.869, -46.8217) -> (21.6697, -46.8217)
  line L1512 (21.6697, -46.8217) -> (21.6697, -45.8227)
  line L1513 (21.6697, -45.8227) -> (35.669, -45.8227)
  line L1514 (35.669, -45.8227) -> (35.669, -46.8217)
  line L1515 (35.669, -46.8217) -> (36.4698, -46.8217)
  line L1516 (36.4698, -46.8217) -> (36.4698, -49.9223)
  line L1517 (36.4698, -49.9223) -> (35.669, -49.9223)
  line L1518 (35.669, -49.9223) -> (35.669, -55.7223)
  line L1519 (35.669, -55.7223) -> (36.4698, -55.7223)
  line L1520 (36.4698, -55.7223) -> (36.4698, -58.8215)
  line L1521 (36.4698, -58.8215) -> (35.669, -58.8215)
  line L1522 (35.669, -58.8215) -> (35.669, -59.8219)
  line L1523 (35.669, -59.8219) -> (21.6697, -59.8219)
  line L1524 (350.282, -74.7723) -> (350.282, -68.9723)
  line L1525 (350.282, -68.9723) -> (349.481, -68.9723)
  line L1526 (349.481, -68.9723) -> (349.481, -65.8717)
  line L1527 (349.481, -65.8717) -> (350.282, -65.8717)
  line L1528 (350.282, -65.8717) -> (350.282, -64.8727)
  line L1529 (350.282, -64.8727) -> (364.282, -64.8727)
  line L1530 (364.282, -64.8727) -> (364.282, -65.8717)
  line L1531 (364.282, -65.8717) -> (365.083, -65.8717)
  line L1532 (365.083, -65.8717) -> (365.083, -68.9723)
  line L1533 (365.083, -68.9723) -> (364.282, -68.9723)
  line L1534 (364.282, -68.9723) -> (364.282, -74.7723)
  line L1535 (364.282, -74.7723) -> (365.083, -74.7723)
  line L1536 (365.083, -74.7723) -> (365.083, -77.8715)
  line L1537 (365.083, -77.8715) -> (364.282, -77.8715)
  line L1538 (364.282, -77.8715) -> (364.282, -78.8719)
  line L1539 (364.282, -78.8719) -> (350.282, -78.8719)
  line L1540 (350.282, -78.8719) -> (350.282, -77.8715)
  line L1541 (350.282, -77.8715) -> (349.481, -77.8715)
  line L1542 (349.481, -77.8715) -> (349.481, -74.7723)
  line L1543 (349.481, -74.7723) -> (350.282, -74.7723)
  line L1544 (302.369, -68.9723) -> (302.369, -74.7723)
  line L1545 (302.369, -74.7723) -> (303.17, -74.7723)
  line L1546 (303.17, -74.7723) -> (303.17, -77.8715)
  line L1547 (303.17, -77.8715) -> (302.369, -77.8715)
  line L1548 (302.369, -77.8715) -> (302.369, -78.8719)
  line L1549 (302.369, -78.8719) -> (288.37, -78.8719)
  line L1550 (288.37, -78.8719) -> (288.37, -77.8715)
  line L1551 (288.37, -77.8715) -> (287.569, -77.8715)
  line L1552 (287.569, -77.8715) -> (287.569, -74.7723)
  line L1553 (287.569, -74.7723) -> (288.37, -74.7723)
  line L1554 (288.37, -74.7723) -> (288.37, -68.9723)
  line L1555 (288.37, -68.9723) -> (287.569, -68.9723)
  line L1556 (287.569, -68.9723) -> (287.569, -65.8717)
  line L1557 (287.569, -65.8717) -> (288.37, -65.8717)
  line L1558 (288.37, -65.8717) -> (288.37, -64.8727)
  line L1559 (288.37, -64.8727) -> (302.369, -64.8727)
  line L1560 (302.369, -64.8727) -> (302.369, -65.8717)
  line L1561 (302.369, -65.8717) -> (303.17, -65.8717)
  line L1562 (303.17, -65.8717) -> (303.17, -68.9723)
  line L1563 (303.17, -68.9723) -> (302.369, -68.9723)
  line L1564 (97.5815, -46.8217) -> (98.3809, -46.8217)
  line L1565 (98.3809, -46.8217) -> (98.3809, -49.9223)
  line L1566 (98.3809, -49.9223) -> (97.5815, -49.9223)
  line L1567 (97.5815, -49.9223) -> (97.5815, -55.7223)
  line L1568 (97.5815, -55.7223) -> (98.3809, -55.7223)
  line L1569 (98.3809, -55.7223) -> (98.3809, -58.8215)
  line L1570 (98.3809, -58.8215) -> (97.5815, -58.8215)
  line L1571 (97.5815, -58.8215) -> (97.5815, -59.8219)
  line L1572 (97.5815, -59.8219) -> (83.5822, -59.8219)
  line L1573 (83.5822, -59.8219) -> (83.5822, -58.8215)
  line L1574 (83.5822, -58.8215) -> (82.7814, -58.8215)
  line L1575 (82.7814, -58.8215) -> (82.7814, -55.7223)
  line L1576 (82.7814, -55.7223) -> (83.5822, -55.7223)
  line L1577 (83.5822, -55.7223) -> (83.5822, -49.9223)
  line L1578 (83.5822, -49.9223) -> (82.7814, -49.9223)
  line L1579 (82.7814, -49.9223) -> (82.7814, -46.8217)
  line L1580 (82.7814, -46.8217) -> (83.5822, -46.8217)
  line L1581 (83.5822, -46.8217) -> (83.5822, -45.8227)
  line L1582 (83.5822, -45.8227) -> (97.5815, -45.8227)
  line L1583 (97.5815, -45.8227) -> (97.5815, -46.8217)
  line L1584 (135.682, -49.9223) -> (135.682, -55.7223)
  line L1585 (135.682, -55.7223) -> (136.481, -55.7223)
  line L1586 (136.481, -55.7223) -> (136.481, -58.8215)
  line L1587 (136.481, -58.8215) -> (135.682, -58.8215)
  line L1588 (135.682, -58.8215) -> (135.682, -59.8219)
  line L1589 (135.682, -59.8219) -> (121.682, -59.8219)
  line L1590 (121.682, -59.8219) -> (121.682, -58.8215)
  line L1591 (121.682, -58.8215) -> (120.881, -58.8215)
  line L1592 (120.881, -58.8215) -> (120.881, -55.7223)
  line L1593 (120.881, -55.7223) -> (121.682, -55.7223)
  line L1594 (121.682, -55.7223) -> (121.682, -49.9223)
  line L1595 (121.682, -49.9223) -> (120.881, -49.9223)
  line L1596 (120.881, -49.9223) -> (120.881, -46.8217)
  line L1597 (120.881, -46.8217) -> (121.682, -46.8217)
  line L1598 (121.682, -46.8217) -> (121.682, -45.8227)
  line L1599 (121.682, -45.8227) -> (135.682, -45.8227)
  line L1600 (135.682, -45.8227) -> (135.682, -46.8217)
  line L1601 (135.682, -46.8217) -> (136.481, -46.8217)
  line L1602 (136.481, -46.8217) -> (136.481, -49.9223)
  line L1603 (136.481, -49.9223) -> (135.682, -49.9223)
  arc A40 (-4.6103, 12.27) -> (-12.6103, 4.27) centre (-4.6103, 4.27) ccw
  line L1604 (-12.6103, 4.27) -> (-12.6104, -105.1519)
  arc A41 (-12.6103, -105.1519) -> (-4.6103, -113.1519) centre (-4.6103, -105.1519) ccw
  line L1605 (-4.6103, -113.1519) -> (371.512, -113.1519)
  arc A42 (371.512, -113.1519) -> (379.512, -105.1519) centre (371.512, -105.1519) ccw
  line L1606 (379.512, -105.1519) -> (379.512, 4.27)
  arc A43 (379.512, 4.27) -> (371.512, 12.27) centre (371.512, 4.27) ccw
  line L1607 (371.512, 12.27) -> (-4.6103, 12.27)
  line L1608 (369.512, -99.1519) -> (369.512, -1.73)
  line L1609 (365.512, 2.27) -> (1.3896, 2.27)
  line L1610 (-2.6103, -1.73) -> (-2.6103, -99.1519)
  line L1611 (169.4884, -103.1519) -> (169.4884, -113.1519)
  line L1612 (154.4884, -103.1519) -> (154.4884, -113.1519)
  line L1613 (379.512, -105.1519) -> (379.512, 4.27)
  arc A44 (379.512, 4.27) -> (371.512, 12.27) centre (371.512, 4.27) ccw
  line L1614 (371.512, 12.27) -> (-4.6103, 12.27)
  arc A45 (-4.6104, 12.27) -> (-12.6103, 4.27) centre (-4.6103, 4.27) ccw
  line L1615 (-12.6103, 4.27) -> (-12.6104, -105.1519)
  arc A46 (-12.6103, -105.1519) -> (-4.6103, -113.1519) centre (-4.6103, -105.1519) ccw
  arc A47 (371.512, -113.1519) -> (379.512, -105.1519) centre (371.512, -105.1519) ccw
  line L1616 (-4.6103, -113.1519) -> (154.4884, -113.1519)
  line L1617 (169.4884, -113.1519) -> (371.512, -113.1519)
  line L1618 (1.3897, -103.1519) -> (154.4884, -103.1519)
  line L1619 (169.4884, -103.1519) -> (365.512, -103.1519)
  arc A48 (-2.6103, -99.1519) -> (1.3897, -103.1519) centre (1.3897, -99.1519) ccw
  arc A49 (1.3897, 2.27) -> (-2.6103, -1.73) centre (1.3897, -1.73) ccw
  arc A50 (369.512, -1.73) -> (365.512, 2.27) centre (365.512, -1.73) ccw
  arc A51 (365.512, -103.1519) -> (369.512, -99.1519) centre (365.512, -99.1519) ccw
  line L1620 (-2.3103, -103.824) -> (-4.6103, -102.4961)
  line L1621 (-4.6103, -102.4961) -> (-6.9103, -103.824)
  line L1622 (-6.9103, -103.824) -> (-6.9103, -106.4798)
  line L1623 (-6.9103, -106.4798) -> (-4.6103, -107.8077)
  line L1624 (-4.6103, -107.8077) -> (-2.3103, -106.4798)
  line L1625 (-2.3103, -106.4798) -> (-2.3103, -103.824)
  line L1626 (-2.3103, 5.5979) -> (-4.6103, 6.9258)
  line L1627 (-4.6103, 6.9258) -> (-6.9103, 5.5979)
  line L1628 (-6.9103, 5.5979) -> (-6.9103, 2.9421)
  line L1629 (-6.9103, 2.9421) -> (-4.6103, 1.6142)
  line L1630 (-4.6103, 1.6142) -> (-2.3103, 2.9421)
  line L1631 (-2.3103, 2.9421) -> (-2.3103, 5.5979)
  line L1632 (373.812, 5.5979) -> (371.512, 6.9258)
  line L1633 (371.512, 6.9258) -> (369.212, 5.5979)
  line L1634 (369.212, 5.5979) -> (369.212, 2.9421)
  line L1635 (369.212, 2.9421) -> (371.512, 1.6142)
  line L1636 (371.512, 1.6142) -> (373.812, 2.9421)
  line L1637 (373.812, 2.9421) -> (373.812, 5.5979)
  line L1638 (373.812, -103.824) -> (371.512, -102.4961)
  line L1639 (371.512, -102.4961) -> (369.212, -103.824)
  line L1640 (369.212, -103.824) -> (369.212, -106.4798)
  line L1641 (369.212, -106.4798) -> (371.512, -107.8077)
  line L1642 (371.512, -107.8077) -> (373.812, -106.4798)
  line L1643 (373.812, -106.4798) -> (373.812, -103.824)
  point P0 (-4.6103, -105.1519)
  point P1 (-4.6103, 4.27)
  point P2 (371.512, 4.27)
  point P3 (371.512, -105.1519)
  dimension "d27" = 15
  dimension "d28" = 167.0988
  dimension "d29" = 4
  dimension "d32" = 2.3
  dimension "d33" = 2.3
  dimension "d34" = 2.3
  dimension "d35" = 2.3
  constraint coincident L1611.start L1618
  constraint coincident L1605 L1611.end
  constraint perpendicular L1605 L1611
  constraint coincident L1605 L1612.end
  constraint perpendicular L1605 L1612
  constraint parallel L1606 L1613
  constraint concentric A43 A44
  constraint parallel L1607 L1614
  constraint concentric A40 A45
  constraint parallel L1604 L1615
  constraint concentric A41 A46
  constraint parallel L1605 L1616
  constraint concentric A42 A47
  constraint tangent L1613 A47
  constraint tangent A47 L1616
  constraint tangent L1613 A44
  constraint tangent A44 L1614
  constraint tangent L1614 A45
  constraint tangent L1615 A46
  constraint tangent A45 L1615
  constraint tangent A46 L1616
  constraint collinear L1616 L1617
  constraint parallel L1606 L1608
  constraint parallel L1607 L1609
  constraint parallel L1604 L1610
  constraint parallel L1605 L1618
  constraint collinear L1618 L1619
  constraint tangent L1610 A48
  constraint tangent L1618 A48
  constraint tangent L1609 A49
  constraint tangent L1610 A49
  constraint equal A48 A49
  constraint tangent L1608 A50
  constraint tangent L1609 A50
  constraint equal A48 A50
  constraint tangent L1608 A51
  constraint tangent L1619 A51
  constraint equal A48 A51
  constraint coincident P0 A36.centre
  constraint coincident P1 A37.centre
  constraint coincident P2 A39.centre
  constraint coincident P3 A38.centre
  measures "d27" distance of L1611 L1612
  measures "d28" distance of L1612 L1615
  measures "d29" radius of A48
  measures "d32" distance of P0 L1625
  measures "d33" distance of P1 L1631
  measures "d34" distance of P2 L1637
  measures "d35" distance of P3 L1643
extrude "Extrude3" add sketch "midlayer" along normal blind 6 separate body contours A40 L1604 A41 L1605 A42 L1606 A43 L1607 L1608 L1609 L1610 L1611 L1612 L1613 A44 L1614 A45 L1615 A46 A47 L1616 L1617 L1618 L1619 A48 A49 A50 A51 makes body 2